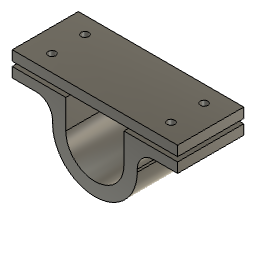
floorcowl_topfloor v17 (Autodesk Fusion 360 design; units mm, degrees)
Autodesk Fusion 360 part; units mm, degrees
note: some values were not read from the file. Set by a fixed rule: which sketch regions a step uses.
sketch "Sketch1" plane through (0, 0, 0) normal (0, 1, 0) x (1, 0, 0)
  circle A0 centre (0, 0) radius 9.525 construction
  line L0 (-25.4, -12.9286) -> (25.4, -12.9286) construction
  line L1 (25.4, -12.9286) -> (25.4, -11.176) construction
  line L2 (25.4, -11.176) -> (-25.4, -11.176) construction
  line L3 (-25.4, -11.176) -> (-25.4, -12.9286) construction
  line L4 (0, -12.9286) -> (0, -11.176)
  line L5 (0, 0) -> (0, -11.176) construction
  line L6 (0, 0) -> (0, -25.4) construction
  line L7 (0, 0) -> (11.176, 0) construction
  line L8 (0, 0) -> (0, 11.176) construction
  line L9 (0, 11.176) -> (0, 16.256)
  line L10 (11.176, 0) -> (11.176, -11.176)
  line L11 (11.176, -11.176) -> (16.256, -11.176)
  line L12 (16.256, -11.176) -> (16.256, 0)
  line L13 (16.256, 0) -> (11.176, 0)
  line L14 (11.176, 0) -> (11.176, -11.176)
  line L15 (0, 0) -> (7.9026, 7.9026) construction
  line L16 (0, 0) -> (11.176, 0) construction
  arc A1 (11.176, 0) -> (0, 11.176) centre (0, 0) ccw
  arc A2 (16.256, 0) -> (0, 16.256) centre (0, 0) ccw
  arc A3 (0, 11.176) -> (-11.176, 0) centre (0, 0) ccw
  arc A4 (0, 16.256) -> (-16.256, 0) centre (0, 0) ccw
  line L17 (-11.176, 0) -> (-11.176, -11.176)
  line L18 (-16.256, -11.176) -> (-16.256, 0)
  line L19 (-11.176, -11.176) -> (-16.256, -11.176)
  line L20 (-16.256, -11.176) -> (-31.75, -11.176)
  line L21 (-31.75, -11.176) -> (-31.75, -7.366)
  line L22 (-31.75, -7.366) -> (-16.256, -7.366)
  line L23 (-16.256, -7.366) -> (-16.256, -11.176)
  line L24 (16.256, -11.176) -> (31.75, -11.176)
  line L25 (31.75, -11.176) -> (31.75, -7.366)
  line L26 (31.75, -7.366) -> (16.256, -7.366)
  line L27 (0, -12.9286) -> (-31.75, -12.9286)
  line L28 (-31.75, -12.9286) -> (-31.75, -16.7386)
  line L29 (-31.75, -16.7386) -> (0, -16.7386)
  line L30 (31.75, -16.7386) -> (0, -16.7386)
  line L31 (31.75, -12.9286) -> (31.75, -16.7386)
  line L32 (0, -12.9286) -> (31.75, -12.9286)
  dimension "d2" = 19.05
  dimension "d3" = 50.8
  dimension "d4" = 1.7526
  dimension "d5" = 1.7526
  dimension "d6" = 25.4
  dimension "d8" = 25.4
  dimension "d12" = 5.08
  dimension "d13" = 5.08
  dimension "d14" = 11.176
  dimension "d15" = 45
  dimension "d16" = 11.176
  dimension "d17" = 11.176
  dimension "d18" = 15.494
  dimension "d19" = 3.81
  dimension "d39" = 11.176
  dimension "d56" = 3.81
  dimension "d57" = 31.75
  constraint coincident A0.centre L5.start
  constraint horizontal L0
  constraint vertical L1
  constraint horizontal L2
  constraint vertical L3
  constraint midpoint L0 L4.start
  constraint midpoint L2 L4.end
  constraint vertical L5
  constraint parallel L5 L6
  constraint perpendicular L5 L7
  constraint perpendicular L7 L8
  constraint parallel L8 L9
  constraint coincident L2 L10.end
  constraint horizontal L11
  constraint vertical L12
  constraint horizontal L13
  constraint vertical L14
  constraint horizontal L16
  constraint coincident L13 L12.end
  constraint symmetric L6 L7.end A3.end
  constraint symmetric L6 L8.end L9.start
  constraint symmetric L6 L9.end A2.end
  constraint symmetric L6 L10.end L17.end
  constraint symmetric L6 L11.end L18.start
  constraint symmetric L6 L12.end A4.end
  constraint symmetric L6 A1 A3
  constraint symmetric L6 A2 A4
  constraint horizontal L20
  constraint vertical L21
  constraint horizontal L22
  constraint vertical L23
  constraint symmetric L6 L18.start L11.end
  constraint symmetric L6 L20.end L24.end
  constraint symmetric L6 L21.end L25.end
  constraint symmetric L6 L22.end L26.end
  constraint perpendicular L4 L27
  constraint perpendicular L27 L28
  constraint coincident L6 L29.end
  constraint perpendicular L6 L29
  constraint symmetric L4.start L6 L27.start
  constraint symmetric L6 L27.end L31.start
  constraint symmetric L6 L28.end L30.start
  constraint symmetric L6 L29.end L30.end
  measures "d2" diameter of A0
  measures "d3" distance of L0.start L0.end
  measures "d4" distance of L0.start L2.end
  measures "d5" distance of L0 L4.end
  measures "d6" distance of L3 L5
  measures "d8" distance of A0.centre L6.end
  measures "d12" distance of L8.end L9.end
  measures "d13" distance of L10.end L11.end
  measures "d14" distance of L10.end L7.end
  measures "d15" angle of L15 L16
  measures "d16" distance of A0.centre L15.end
  measures "d17" distance of A0.centre L7.end
  measures "d18" distance of L18.start L20.end
  measures "d19" distance of L18.start L22.end
  measures "d39" radius of A3
  measures "d56" distance of L27.end L28.end
  measures "d57" distance of L4.start L27.end
extrude "Extrude1" add sketch "Sketch1" along normal blind 25.4 contours L9 A3 A4 L17 L18 L19 L23 | L9 L13 A1 A2 | L10 L11 L12 L13 L14 | L12 L24 L25 L26 | L18 L20 L21 L22 L23 makes body 1
fillet "Fillet1" radius 6.35 2 edges at (16.256, 12.7, 7.366) (-16.256, 12.7, 7.366) on bodies 1
extrude "Extrude2" add sketch "Sketch1" along normal blind 25.4 separate body contours L27 L28 L29 L30 L31 L32 makes body 2
sketch "Sketch5" plane through (0, 0, 16.7386) normal (0, 0, 1) x (-1, 0, 0)
  line L0 (31.75, 0) -> (-31.75, 0)
  line L1 (-31.75, 0) -> (-31.75, -25.4)
  line L2 (-31.75, -25.4) -> (31.75, -25.4)
  line L3 (31.75, -25.4) -> (31.75, 0)
  line L4 (31.75, -25.4) -> (-31.75, -25.4) construction
  line L5 (-31.75, -25.4) -> (-31.75, 0) construction
  line L6 (-31.75, 0) -> (31.75, 0) construction
  line L7 (31.75, 0) -> (31.75, -25.4) construction
  line L8 (0, -25.4) -> (0, 0) construction
  line L9 (-22.86, 0) -> (-22.86, -25.4) construction
  line L10 (-22.86, -12.7) -> (0, -12.7) construction
  line L11 (-22.86, -19.05) -> (0, -19.05) construction
  line L12 (0, -6.35) -> (-22.86, -6.35) construction
  point P0 (-22.86, -19.05)
  point P1 (-22.86, -6.35)
  point P2 (22.86, -19.05)
  point P3 (22.86, -6.35)
  dimension "d60" = 8.89
  dimension "d61" = 6.35
  dimension "d62" = 6.35
  constraint horizontal L4
  constraint vertical L5
  constraint horizontal L6
  constraint vertical L7
  constraint coincident L0.end L1.start
  constraint coincident L2.end L3.start
  constraint midpoint L4 L8.start
  constraint coincident L8.end origin
  constraint coincident L0 L9.start
  constraint coincident L2 L9.end
  constraint perpendicular L2 L9
  constraint midpoint L9 L10.start
  constraint midpoint L8 L10.end
  constraint coincident L9 P0
  constraint coincident L8 L11.end
  constraint perpendicular L8 L11
  constraint coincident L8 L12.start
  constraint coincident L9 P1
  constraint perpendicular L9 L12
  constraint coincident P0 L11.start
  constraint coincident P1 L12.end
  constraint symmetric L8 P0 P2
  constraint symmetric L8 P1 P3
  measures "d60" distance of L5 L9
  measures "d61" distance of L4 L11
  measures "d62" distance of L6 L12
hole "Hole6" at (-22.86, 19.05, 16.7386) at (-22.86, 6.35, 16.7386) at (22.86, 19.05, 16.7386) at (22.86, 6.35, 16.7386) direction (0, 0, -1) diameter 2.8702 depth 11.1252 tip angle 180 bodies 1 2
